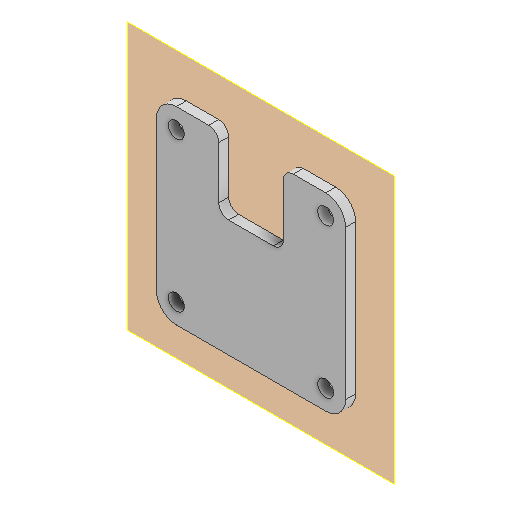
# Autodesk Inventor part: 20_Cube_Insert_SEEED_Xiao_Sense_Camera_backplate_inplate
Saved by Autodesk Inventor 2022 (Build 260153000, 153)
## iProperties
Created: 2023-04-27
Part Number: 20_Cube_Insert_SEEED_Xiao_Sense_Camera_backplate_inplate
Material: Generisch
Document SubType Name: Modeling
Designer: diederichbenedict
Density: 1 g/cm^3
Appearance: Vorgabe
Author: diederichbenedict
Autodesk Inventor part; units mm, degrees
ref_plane "YZ Plane" through (0, 0, 0) normal (1, 0, 0) x (0, 1, 0)
ref_plane "XZ Plane" through (0, 0, 0) normal (0, 1, 0) x (-1, 0, 0)
ref_plane "XY Plane" through (0, 0, 0) normal (0, 0, 1) x (1, 0, 0)
ref_plane "Arbeitsebene1" through (0, 0, 0) normal (0, 0, 1) x (1, 0, 0)
sketch "Skizze1" plane through (0, 0, 0) normal (0, 0, 1) x (1, 0, 0)
  line L0 (8.0712, 15) -> (38.0712, 15)
  line L1 (38.0712, 15) -> (38.0712, -15)
  line L2 (38.0712, -15) -> (8.0712, -15)
  line L3 (8.0712, -15) -> (8.0712, 15)
  line L4 (38.0712, 19) -> (8.0712, 19)
  line L5 (4.0712, 15) -> (4.0712, -15)
  line L6 (8.0712, -19) -> (38.0712, -19)
  line L7 (42.0712, -15) -> (42.0712, 15)
  arc A0 (8.0712, 19) -> (4.0712, 15) centre (8.0712, 15) ccw
  arc A1 (42.0712, 15) -> (38.0712, 19) centre (38.0712, 15) ccw
  arc A2 (38.0712, -19) -> (42.0712, -15) centre (38.0712, -15) ccw
  arc A3 (4.0712, -15) -> (8.0712, -19) centre (8.0712, -15) ccw
  line L8 (29.9712, -18.3074) -> (29.9712, -24.4) projected
  circle A4 centre (38.0712, -15) radius 1.4 projected
  circle A5 centre (38.0712, 15) radius 1.4 projected
  line L9 (39.5712, -24.4) -> (29.9712, -24.4) projected
  line L10 (39.5712, -21.1181) -> (39.5712, -24.4) projected
  line L11 (44.1893, -16.5) -> (39.5712, -21.1181) projected
  line L12 (47.4712, -16.5) -> (44.1893, -16.5) projected
  line L13 (47.4712, 16.5) -> (47.4712, -16.5) projected
  line L14 (44.1893, 16.5) -> (47.4712, 16.5) projected
  line L15 (39.5712, 21.1181) -> (44.1893, 16.5) projected
  line L16 (39.5712, 24.4) -> (39.5712, 21.1181) projected
  line L17 (31.5712, 24.4) -> (39.5712, 24.4) projected
  line L18 (31.5712, 4.0068) -> (31.5712, 24.4) projected
  arc A6 (32.7786, 1.7) -> (31.5712, 4.0068) centre (29.9712, 1.7) ccw projected
  line L19 (32.7786, 1.7) -> (32.7786, -15.5) projected
  arc A7 (29.9712, -18.3074) -> (32.7786, -15.5) centre (29.9712, -15.5) ccw projected
  point P0 (0, 0)
  point P1 (36.5793, -24.4)
  point P2 (31.5712, 11.3758)
  dimension "d0" = 4
  dimension "d1" = 4
  constraints: 16 end point, 8 point on circle, 8 tangent, 4 centre point, 4 parallel, 3 equal radius, 2 perpendicular, 1 horizontal, 3 other
  measures "d0" distance between parallel lines of L0 L4
  measures "d1" radius of A0
extrude "Extrusion1" add sketch "Skizze1" along normal blind 2 contours L3 L2 L19 A7 L8 L6 A3 L5 A0 L4 L18 L0 | L0 L18 A6 L19 L2 L3 | L18 L4 A1 L7 A2 L6 L8 A7 L19 L2 A4 L1 A5 L0 | L0 A5 L1 A4 L2 L19 A6 L18 | A5 L1 L0 | L0 L1 A5 | A4 L1 L2 | L2 L1 A4
ref_plane "Arbeitsebene2" through (0, 0, 0) normal (0, 0, 1) x (1, 0, 0)
sketch "Skizze2" plane through (0, 0, 2) normal (0, 0, 1) x (1, 0, 0)
  arc A0 (8.0712, 19) -> (4.0712, 15) centre (8.0712, 15) ccw projected
  line L0 (4.0712, 15) -> (4.0712, -15) projected
  arc A1 (4.0712, -15) -> (8.0712, -19) centre (8.0712, -15) ccw projected
  line L1 (8.0712, -19) -> (38.0712, -19) projected
  arc A2 (38.0712, -19) -> (42.0712, -15) centre (38.0712, -15) ccw projected
  line L2 (42.0712, -15) -> (42.0712, 15) projected
  arc A3 (42.0712, 15) -> (38.0712, 19) centre (38.0712, 15) ccw projected
  line L3 (38.0712, 19) -> (8.0712, 19) projected
  circle A4 centre (8.0712, 15) radius 1.4 projected
  circle A5 centre (38.0712, 15) radius 1.4 projected
  circle A6 centre (38.0712, -15) radius 1.4 projected
  circle A7 centre (8.0712, -15) radius 1.4 projected
  point P0 (0, 0)
hole "Bohrung1" at (8.0712, 15, 2) at (8.0712, -15, 2) at (38.0712, -15, 2) at (38.0712, 15, 2) direction (0, 0, -1) diameter 3.2 end through all
sketch "Skizze3" plane through (0, 0, 2) normal (0, 0, 1) x (1, 0, 0)
  circle A0 centre (23.0919, -0.0207) radius 4.25 projected
  arc A1 (30.2483, 24.4) -> (29.5712, 22.9) centre (31.5712, 22.9) ccw projected
  line L0 (39.5712, 24.4) -> (30.2483, 24.4) projected
  line L1 (39.5712, 21.1181) -> (39.5712, 24.4) projected
  line L2 (44.1893, 16.5) -> (39.5712, 21.1181) projected
  line L3 (47.4712, 16.5) -> (44.1893, 16.5) projected
  line L4 (47.4712, -16.5) -> (47.4712, 16.5) projected
  line L5 (44.1893, -16.5) -> (47.4712, -16.5) projected
  line L6 (39.5712, -21.1181) -> (44.1893, -16.5) projected
  line L7 (39.5712, -24.4) -> (39.5712, -21.1181) projected
  line L8 (6.6126, -24.4) -> (39.5712, -24.4) projected
  line L9 (6.6126, -21.1595) -> (6.6126, -24.4) projected
  line L10 (1.9531, -16.5) -> (6.6126, -21.1595) projected
  line L11 (-1.3288, -16.5) -> (1.9531, -16.5) projected
  line L12 (-1.3288, 16.5) -> (-1.3288, -16.5) projected
  line L13 (1.9531, 16.5) -> (-1.3288, 16.5) projected
  line L14 (6.5712, 21.1181) -> (1.9531, 16.5) projected
  line L15 (6.5712, 24.4) -> (6.5712, 21.1181) projected
  line L16 (15.894, 24.4) -> (6.5712, 24.4) projected
  arc A2 (16.5712, 22.9) -> (15.894, 24.4) centre (14.5712, 22.9) ccw projected
  line L17 (16.5712, 22.9) -> (16.5712, 6.5074) projected
  arc A3 (16.5712, 6.5074) -> (18.5712, 4.5074) centre (18.5712, 6.5074) ccw projected
  line L18 (18.5712, 4.5074) -> (27.5712, 4.5074) projected
  arc A4 (27.5712, 4.5074) -> (29.5712, 6.5074) centre (27.5712, 6.5074) ccw projected
  line L19 (29.5712, 6.5074) -> (29.5712, 22.9) projected
  circle A5 centre (38.0712, 15) radius 1.4 projected
  circle A6 centre (8.0712, -15) radius 1.4 projected
  circle A7 centre (38.0712, -15) radius 1.4 projected
  circle A8 centre (8.0712, 15) radius 1.4 projected
  line L20 (15.894, 24.4) -> (30.2483, 24.4)
  point P0 (0, 0)
  constraints: 2 end point, 1 horizontal
extrude "Extrusion2" cut sketch "Skizze3" against normal blind 10 contours A1 L19 A4 L18 A3 L17 A2 L20
fillet "Rundung1" radius 2 2 edges at (16.5712, 19, 1) (29.5712, 19, 1)
